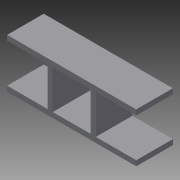
# Autodesk Inventor part: Parametric
Saved by Autodesk Inventor 2015 (Build 190159000, 159)
## iProperties
Created: 2017-01-04
Part Number: Parametric
Material: Generic
Document SubType Name: Modeling
Designer: Rudge-Top
Density: 1 g/cm^3
Appearance: Default
Author: Rudge-Top
Autodesk Inventor part; units mm, degrees
ref_plane "YZ Plane" through (0, 0, 0) normal (1, 0, 0) x (0, 1, 0)
ref_plane "XZ Plane" through (0, 0, 0) normal (0, 1, 0) x (-1, 0, 0)
ref_plane "XY Plane" through (0, 0, 0) normal (0, 0, 1) x (1, 0, 0)
sketch "Sketch1" plane through (0, 0, 0) normal (0, 1, 0) x (-1, 0, 0)
  line L0 (0, 0) -> (123.5, 0)
  line L1 (123.5, 0) -> (123.5, -5)
  line L2 (123.5, -5) -> (0, -5)
  line L3 (0, -5) -> (0, 0)
  line L4 (0, -47.1) -> (123.5, -47.1)
  line L5 (123.5, -47.1) -> (123.5, -42.1)
  line L6 (123.5, -42.1) -> (0, -42.1)
  line L7 (0, -42.1) -> (0, -47.1)
  dimension "d0" = 123.5
  dimension "d1" = 5
  dimension "d2" = 123.5
  dimension "d3" = 5
  dimension "d4" = 47.1
  dimension "d7" = 0
  constraints: 16 end point, 4 parallel, 2 horizontal, 2 perpendicular
  measures "d0" distance of L1.end L2.end
  measures "d1" distance of L0.end L1.end
  measures "d2" distance of L6.end L5.end
  measures "d3" distance of L5.end L4.end
  measures "d4" distance between parallel lines of L4 L0
  measures "d7" distance between parallel lines of L3 L7
extrude "Extrusion1" add sketch "Sketch1" along normal blind 35
sketch "Sketch2" plane through (0, 35, 0) normal (0, 1, 0) x (1, 0, 0)
  line L0 (-123.5, 0) -> (0, 0) projected
  line L1 (0, 0) -> (0, 5) projected
  line L2 (0, 5) -> (-123.5, 5) projected
  line L3 (-123.5, 5) -> (-123.5, 0) projected
  line L4 (0, 47.1) -> (-123.5, 47.1) projected
  line L5 (-123.5, 47.1) -> (-123.5, 42.1) projected
  line L6 (-123.5, 42.1) -> (0, 42.1) projected
  line L7 (0, 42.1) -> (0, 47.1) projected
  line L8 (-38.6667, 5) -> (-43.6667, 5)
  line L9 (-43.6667, 5) -> (-43.6667, 42.1)
  line L10 (-43.6667, 42.1) -> (-38.6667, 42.1)
  line L11 (-38.6667, 42.1) -> (-38.6667, 5)
  line L12 (-123.5, 42.1) -> (0, 42.1) projected
  line L13 (-84.8333, 5) -> (-79.8333, 5)
  line L14 (-79.8333, 5) -> (-79.8333, 42.1)
  line L15 (-79.8333, 42.1) -> (-84.8333, 42.1)
  line L16 (-84.8333, 42.1) -> (-84.8333, 5)
  dimension "d8" = 5
  dimension "d9" = 5
  dimension "d10" = 38.6667
  dimension "d11" = 38.6667
  constraints: 16 end point, 4 parallel, 4 point on line, 2 horizontal, 2 perpendicular
  measures "d8" distance of L9.end L10.end
  measures "d9" distance of L15.end L14.end
  measures "d10" distance between parallel lines of L1 L11
  measures "d11" distance between parallel lines of L3 L16
extrude "Extrusion2" add sketch "Sketch2" against normal blind 35 contours L16 L6 L14 L2 | L2 L9 L6 L11
body "Solid1"
